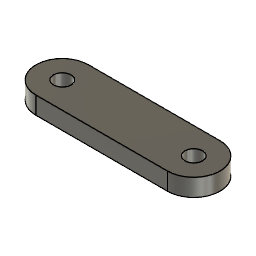
Gear_Reduction_System_V2 (Autodesk Fusion 360 archive; units mm, degrees)
design "Base_Plate"
part number: 2026-07-07-20-07-20-586
Autodesk Fusion 360 part; units mm, degrees
sketch "Sketch1" plane through (0, 0, 0) normal (0, 0, 1) x (1, 0, 0)
  line L0 (0, -15) -> (75, -15)
  arc A0 (75, -15) -> (75, 15) centre (75, 0) ccw
  line L1 (75, 15) -> (0, 15)
  arc A1 (0, 15) -> (0, -15) centre (0, 0) ccw
  line L2 (0, 0) -> (75, 0) construction
  circle A2 centre (0, 0) radius 5
  circle A3 centre (75, 0) radius 5
  dimension "d1" = 30
  dimension "d2" = 10
  dimension "d3" = 10
  dimension "d4" = 75
  constraint tangent L0 A0
  constraint tangent A0 L1
  constraint parallel L0 L1
  constraint tangent L1 A1
  constraint tangent L0 A1
  constraint horizontal L2
  constraint coincident A1.centre L2.start
  constraint concentric A0 A3
  measures "d1" diameter of A0
  measures "d2" diameter of A2
  measures "d3" diameter of A3
  measures "d4" distance of A1.centre A0.centre
extrude "Extrude1" add sketch "Sketch1" against normal blind 10

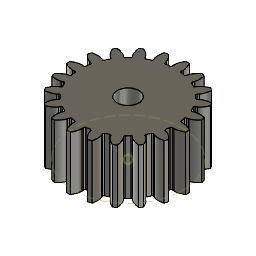
design "Input_Pinion_V2_locked"
description: Spur Gear; Module: 2.5; Num Teeth: 20; Pressure Angle: 20.0; Backlash: 0.10 mm
part number: 2026-07-07-19-52-48-720
Autodesk Fusion 360 part; units mm, degrees
sketch "Base Circle" plane through (0, 0, 0) normal (0, 0, 1) x (1, 0, 0)
  circle A0 centre (0, 0) radius 22.1075
  circle A1 centre (0, 0) radius 5
extrude "Extrude1" add sketch "Base Circle" along normal blind 25
sketch "Gear Tooth" plane through (0, 0, 0) normal (0, 0, 1) x (1, 0, 0)
  spline S0 degree 5 poles (23.392, -2.1686) (23.4038, -2.1697) (23.4273, -2.1716) (23.4626, -2.1735) (23.5098, -2.1741) (23.5688, -2.1726) (23.6279, -2.1692) (23.6871, -2.1648) (23.7463, -2.1597) (23.8055, -2.1543) (23.8647, -2.1485) (23.924, -2.1421) (23.9832, -2.135) (24.0425, -2.127) (24.1018, -2.1182) (24.161, -2.1085) (24.2203, -2.0982) (24.2796, -2.0873) (24.3388, -2.076) (24.3981, -2.0641) (24.4573, -2.0518) (24.5166, -2.039) (24.5758, -2.0257) (24.635, -2.0118) (24.6941, -1.9974) (24.7533, -1.9825) (24.8124, -1.9672) (24.8715, -1.9513) (24.9306, -1.935) (24.9897, -1.9183) (25.0487, -1.9012) (25.1077, -1.8836) (25.1666, -1.8656) (25.2256, -1.8472) (25.2845, -1.8283) (25.3433, -1.809) (25.4022, -1.7894) (25.461, -1.7693) (25.5197, -1.7488) (25.5784, -1.7279) (25.6371, -1.7067) (25.6957, -1.6851) (25.7543, -1.663) (25.8129, -1.6407) (25.8714, -1.6179) (25.9298, -1.5948) (25.9882, -1.5713) (26.0466, -1.5474) (26.1049, -1.5232) (26.1632, -1.4986) (26.2214, -1.4737) (26.2795, -1.4484) (26.3376, -1.4228) (26.3957, -1.3968) (26.4537, -1.3705) (26.5116, -1.3438) (26.5695, -1.3169) (26.6273, -1.2895) (26.6851, -1.2619) (26.7428, -1.2339) (26.8004, -1.2056) (26.858, -1.1769) (26.9155, -1.148) (26.973, -1.1187) (27.0304, -1.0891) (27.0877, -1.0592) (27.145, -1.029) (27.2022, -0.9984) (27.2593, -0.9676) (27.3164, -0.9364) (27.3734, -0.9049) (27.4189, -0.8795) (27.453, -0.8603) (27.4758, -0.8474) (27.4871, -0.841) knots 0 0 0 0 0 0 0.01428571 0.02857143 0.04285714 0.05714286 0.07142857 0.08571429 0.1 0.11428571 0.12857143 0.14285714 0.15714286 0.17142857 0.18571429 0.2 0.21428571 0.22857143 0.24285714 0.25714286 0.27142857 0.28571429 0.3 0.31428571 0.32857143 0.34285714 0.35714286 0.37142857 0.38571429 0.4 0.41428571 0.42857143 0.44285714 0.45714286 0.47142857 0.48571429 0.5 0.51428571 0.52857143 0.54285714 0.55714286 0.57142857 0.58571429 0.6 0.61428571 0.62857143 0.64285714 0.65714286 0.67142857 0.68571429 0.7 0.71428571 0.72857143 0.74285714 0.75714286 0.77142857 0.78571429 0.8 0.81428571 0.82857143 0.84285714 0.85714286 0.87142857 0.88571429 0.9 0.91428571 0.92857143 0.94285714 0.95714286 0.97142857 0.98571429 1 1 1 1 1 1
  spline S1 degree 5 poles (23.392, 2.1686) (23.4038, 2.1697) (23.4273, 2.1716) (23.4626, 2.1735) (23.5098, 2.1741) (23.5688, 2.1726) (23.6279, 2.1692) (23.6871, 2.1648) (23.7463, 2.1597) (23.8055, 2.1543) (23.8647, 2.1485) (23.924, 2.1421) (23.9832, 2.135) (24.0425, 2.127) (24.1018, 2.1182) (24.161, 2.1085) (24.2203, 2.0982) (24.2796, 2.0873) (24.3388, 2.076) (24.3981, 2.0641) (24.4573, 2.0518) (24.5166, 2.039) (24.5758, 2.0257) (24.635, 2.0118) (24.6941, 1.9974) (24.7533, 1.9825) (24.8124, 1.9672) (24.8715, 1.9513) (24.9306, 1.935) (24.9897, 1.9183) (25.0487, 1.9012) (25.1077, 1.8836) (25.1666, 1.8656) (25.2256, 1.8472) (25.2845, 1.8283) (25.3433, 1.809) (25.4022, 1.7894) (25.461, 1.7693) (25.5197, 1.7488) (25.5784, 1.7279) (25.6371, 1.7067) (25.6957, 1.6851) (25.7543, 1.663) (25.8129, 1.6407) (25.8714, 1.6179) (25.9298, 1.5948) (25.9882, 1.5713) (26.0466, 1.5474) (26.1049, 1.5232) (26.1632, 1.4986) (26.2214, 1.4737) (26.2795, 1.4484) (26.3376, 1.4228) (26.3957, 1.3968) (26.4537, 1.3705) (26.5116, 1.3438) (26.5695, 1.3169) (26.6273, 1.2895) (26.6851, 1.2619) (26.7428, 1.2339) (26.8004, 1.2056) (26.858, 1.1769) (26.9155, 1.148) (26.973, 1.1187) (27.0304, 1.0891) (27.0877, 1.0592) (27.145, 1.029) (27.2022, 0.9984) (27.2593, 0.9676) (27.3164, 0.9364) (27.3734, 0.9049) (27.4189, 0.8795) (27.453, 0.8603) (27.4758, 0.8474) (27.4871, 0.841) knots 0 0 0 0 0 0 0.01428571 0.02857143 0.04285714 0.05714286 0.07142857 0.08571429 0.1 0.11428571 0.12857143 0.14285714 0.15714286 0.17142857 0.18571429 0.2 0.21428571 0.22857143 0.24285714 0.25714286 0.27142857 0.28571429 0.3 0.31428571 0.32857143 0.34285714 0.35714286 0.37142857 0.38571429 0.4 0.41428571 0.42857143 0.44285714 0.45714286 0.47142857 0.48571429 0.5 0.51428571 0.52857143 0.54285714 0.55714286 0.57142857 0.58571429 0.6 0.61428571 0.62857143 0.64285714 0.65714286 0.67142857 0.68571429 0.7 0.71428571 0.72857143 0.74285714 0.75714286 0.77142857 0.78571429 0.8 0.81428571 0.82857143 0.84285714 0.85714286 0.87142857 0.88571429 0.9 0.91428571 0.92857143 0.94285714 0.95714286 0.97142857 0.98571429 1 1 1 1 1 1
  arc A0 (27.4871, -0.841) -> (27.4871, 0.841) centre (0, 0) ccw
  line L0 (22.0031, -2.0399) -> (23.392, -2.1686)
  line L1 (22.0031, 2.0399) -> (23.392, 2.1686)
  line L2 (22.0031, -2.0399) -> (22.0031, 2.0399)
  point P0 (23.6798, -2.1652)
  point P1 (23.9698, -2.1364)
  point P2 (24.2612, -2.0907)
  point P3 (24.5535, -2.0306)
  point P4 (24.8466, -1.9579)
  point P5 (25.1402, -1.8736)
  point P6 (25.4341, -1.7784)
  point P7 (25.7281, -1.6729)
  point P8 (26.0221, -1.5574)
  point P9 (26.316, -1.4323)
  point P10 (26.6096, -1.2979)
  point P11 (26.9027, -1.1544)
  point P12 (27.1953, -1.002)
  point P13 (23.6798, 2.1652)
  point P14 (23.9698, 2.1364)
  point P15 (24.2612, 2.0907)
  point P16 (24.5535, 2.0306)
  point P17 (24.8466, 1.9579)
  point P18 (25.1402, 1.8736)
  point P19 (25.4341, 1.7784)
  point P20 (25.7281, 1.6729)
  point P21 (26.0221, 1.5574)
  point P22 (26.316, 1.4323)
  point P23 (26.6096, 1.2979)
  point P24 (26.9027, 1.1544)
  point P25 (27.1953, 1.002)
extrude "Extrude2" add sketch "Gear Tooth" along normal blind 25
fillet "Fillet1" radius 0.5 2 edges at (22.0131, -2.0408, 12.5) (22.0131, 2.0408, 12.5)
pattern_circular "C-Pattern1" count 20 over 360 about axis through (0, 0, 0) along (0, 0, 1) of "Extrude2", "Fillet1"
sketch "Diametrial Pitch Circle" plane through (0, 0, 0) normal (0, 0, 1) x (1, 0, 0)
  circle A0 centre (0, 0) radius 25 construction

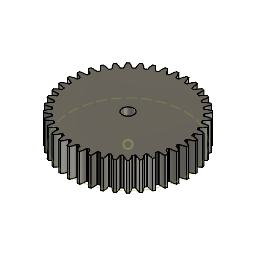
design "Output_Gear_V2_locked"
description: Spur Gear; Module: 2.5; Num Teeth: 40; Pressure Angle: 20.0; Backlash: 0.10 mm
part number: 2026-07-07-19-55-07-887
Autodesk Fusion 360 part; units mm, degrees
sketch "Base Circle" plane through (0, 0, 0) normal (0, 0, 1) x (1, 0, 0)
  circle A0 centre (0, 0) radius 47.1075
  circle A1 centre (0, 0) radius 5
extrude "Extrude1" add sketch "Base Circle" along normal blind 25
sketch "Gear Tooth" plane through (0, 0, 0) normal (0, 0, 1) x (1, 0, 0)
  spline S0 degree 5 poles (46.917, -2.5207) (46.9331, -2.5208) (46.9653, -2.5209) (47.0136, -2.5207) (47.078, -2.5196) (47.1586, -2.5168) (47.2392, -2.5128) (47.3198, -2.5074) (47.4004, -2.5008) (47.481, -2.4931) (47.5617, -2.4844) (47.6423, -2.4747) (47.7229, -2.4643) (47.8035, -2.4531) (47.8841, -2.4413) (47.9646, -2.4289) (48.0451, -2.4157) (48.1257, -2.402) (48.2061, -2.3875) (48.2866, -2.3725) (48.3671, -2.3568) (48.4475, -2.3405) (48.5279, -2.3237) (48.6082, -2.3063) (48.6885, -2.2884) (48.7688, -2.27) (48.8491, -2.2511) (48.9293, -2.2316) (49.0095, -2.2117) (49.0896, -2.1913) (49.1698, -2.1703) (49.2498, -2.1489) (49.3299, -2.1271) (49.4099, -2.1047) (49.4899, -2.0819) (49.5698, -2.0587) (49.6497, -2.0351) (49.7295, -2.011) (49.8093, -1.9864) (49.889, -1.9615) (49.9687, -1.9361) (50.0484, -1.9103) (50.128, -1.8841) (50.2076, -1.8575) (50.2871, -1.8305) (50.3666, -1.8031) (50.446, -1.7753) (50.5254, -1.7471) (50.6047, -1.7185) (50.684, -1.6895) (50.7632, -1.6602) (50.8424, -1.6305) (50.9215, -1.6004) (51.0006, -1.5699) (51.0796, -1.5391) (51.1585, -1.5079) (51.2374, -1.4764) (51.3163, -1.4445) (51.3951, -1.4122) (51.4738, -1.3796) (51.5525, -1.3466) (51.6311, -1.3133) (51.7096, -1.2796) (51.7881, -1.2456) (51.8666, -1.2113) (51.945, -1.1766) (52.0233, -1.1416) (52.1015, -1.1063) (52.1797, -1.0706) (52.2579, -1.0346) (52.3359, -0.9983) (52.3983, -0.9689) (52.4451, -0.9468) (52.4763, -0.932) (52.4919, -0.9245) knots 0 0 0 0 0 0 0.01428571 0.02857143 0.04285714 0.05714286 0.07142857 0.08571429 0.1 0.11428571 0.12857143 0.14285714 0.15714286 0.17142857 0.18571429 0.2 0.21428571 0.22857143 0.24285714 0.25714286 0.27142857 0.28571429 0.3 0.31428571 0.32857143 0.34285714 0.35714286 0.37142857 0.38571429 0.4 0.41428571 0.42857143 0.44285714 0.45714286 0.47142857 0.48571429 0.5 0.51428571 0.52857143 0.54285714 0.55714286 0.57142857 0.58571429 0.6 0.61428571 0.62857143 0.64285714 0.65714286 0.67142857 0.68571429 0.7 0.71428571 0.72857143 0.74285714 0.75714286 0.77142857 0.78571429 0.8 0.81428571 0.82857143 0.84285714 0.85714286 0.87142857 0.88571429 0.9 0.91428571 0.92857143 0.94285714 0.95714286 0.97142857 0.98571429 1 1 1 1 1 1
  spline S1 degree 5 poles (46.917, 2.5207) (46.9331, 2.5208) (46.9653, 2.5209) (47.0136, 2.5207) (47.078, 2.5196) (47.1586, 2.5168) (47.2392, 2.5128) (47.3198, 2.5074) (47.4004, 2.5008) (47.481, 2.4931) (47.5617, 2.4844) (47.6423, 2.4747) (47.7229, 2.4643) (47.8035, 2.4531) (47.8841, 2.4413) (47.9646, 2.4289) (48.0451, 2.4157) (48.1257, 2.402) (48.2061, 2.3875) (48.2866, 2.3725) (48.3671, 2.3568) (48.4475, 2.3405) (48.5279, 2.3237) (48.6082, 2.3063) (48.6885, 2.2884) (48.7688, 2.27) (48.8491, 2.2511) (48.9293, 2.2316) (49.0095, 2.2117) (49.0896, 2.1913) (49.1698, 2.1703) (49.2498, 2.1489) (49.3299, 2.1271) (49.4099, 2.1047) (49.4899, 2.0819) (49.5698, 2.0587) (49.6497, 2.0351) (49.7295, 2.011) (49.8093, 1.9864) (49.889, 1.9615) (49.9687, 1.9361) (50.0484, 1.9103) (50.128, 1.8841) (50.2076, 1.8575) (50.2871, 1.8305) (50.3666, 1.8031) (50.446, 1.7753) (50.5254, 1.7471) (50.6047, 1.7185) (50.684, 1.6895) (50.7632, 1.6602) (50.8424, 1.6305) (50.9215, 1.6004) (51.0006, 1.5699) (51.0796, 1.5391) (51.1585, 1.5079) (51.2374, 1.4764) (51.3163, 1.4445) (51.3951, 1.4122) (51.4738, 1.3796) (51.5525, 1.3466) (51.6311, 1.3133) (51.7096, 1.2796) (51.7881, 1.2456) (51.8666, 1.2113) (51.945, 1.1766) (52.0233, 1.1416) (52.1015, 1.1063) (52.1797, 1.0706) (52.2579, 1.0346) (52.3359, 0.9983) (52.3983, 0.9689) (52.4451, 0.9468) (52.4763, 0.932) (52.4919, 0.9245) knots 0 0 0 0 0 0 0.01428571 0.02857143 0.04285714 0.05714286 0.07142857 0.08571429 0.1 0.11428571 0.12857143 0.14285714 0.15714286 0.17142857 0.18571429 0.2 0.21428571 0.22857143 0.24285714 0.25714286 0.27142857 0.28571429 0.3 0.31428571 0.32857143 0.34285714 0.35714286 0.37142857 0.38571429 0.4 0.41428571 0.42857143 0.44285714 0.45714286 0.47142857 0.48571429 0.5 0.51428571 0.52857143 0.54285714 0.55714286 0.57142857 0.58571429 0.6 0.61428571 0.62857143 0.64285714 0.65714286 0.67142857 0.68571429 0.7 0.71428571 0.72857143 0.74285714 0.75714286 0.77142857 0.78571429 0.8 0.81428571 0.82857143 0.84285714 0.85714286 0.87142857 0.88571429 0.9 0.91428571 0.92857143 0.94285714 0.95714286 0.97142857 0.98571429 1 1 1 1 1 1
  arc A0 (52.4919, -0.9245) -> (52.4919, 0.9245) centre (0, 0) ccw
  line L0 (46.917, 2.5207) -> (46.917, -2.5207)
  point P0 (47.3122, -2.5077)
  point P1 (47.7089, -2.466)
  point P2 (48.1064, -2.4051)
  point P3 (48.5046, -2.3285)
  point P4 (48.9032, -2.2379)
  point P5 (49.3022, -2.1346)
  point P6 (49.7013, -2.0194)
  point P7 (50.1005, -1.8931)
  point P8 (50.4997, -1.7561)
  point P9 (50.8988, -1.609)
  point P10 (51.2976, -1.452)
  point P11 (51.6961, -1.2854)
  point P12 (52.0942, -1.1095)
  point P13 (47.3122, 2.5077)
  point P14 (47.7089, 2.466)
  point P15 (48.1064, 2.4051)
  point P16 (48.5046, 2.3285)
  point P17 (48.9032, 2.2379)
  point P18 (49.3022, 2.1346)
  point P19 (49.7013, 2.0194)
  point P20 (50.1005, 1.8931)
  point P21 (50.4997, 1.7561)
  point P22 (50.8988, 1.609)
  point P23 (51.2976, 1.452)
  point P24 (51.6961, 1.2854)
  point P25 (52.0942, 1.1095)
extrude "Extrude2" add sketch "Gear Tooth" along normal blind 25
fillet "Fillet1" radius 0.5 2 edges at (47.04, 2.5201, 12.5) (47.04, -2.5201, 12.5)
pattern_circular "C-Pattern1" count 40 over 360 about axis through (0, 0, 0) along (0, 0, 1) of "Extrude2", "Fillet1"
sketch "Diametrial Pitch Circle" plane through (0, 0, 0) normal (0, 0, 1) x (1, 0, 0)
  circle A0 centre (0, 0) radius 50 construction
